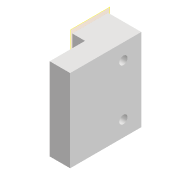
# Autodesk Inventor part: 30_XYTable_Aliexpress_Translatorarm_y
Saved by Autodesk Inventor 2022 (Build 260153000, 153)
## iProperties
Created: 2022-10-26
Part Number: 30_XYTable_Aliexpress_Translatorarm_y
Material: Generisch
Document SubType Name: Modeling
Designer: diederichbenedict
Density: 1 g/cm^3
Appearance: Vorgabe
Author: diederichbenedict
Autodesk Inventor part; units mm, degrees
ref_plane "YZ Plane" through (0, 0, 0) normal (1, 0, 0) x (0, 1, 0)
ref_plane "XZ Plane" through (0, 0, 0) normal (0, 1, 0) x (-1, 0, 0)
ref_plane "XY Plane" through (0, 0, 0) normal (0, 0, 1) x (1, 0, 0)
ref_plane "Arbeitsebene2" through (35, 26.0506, 0) normal (1, 0, 0) x (0, 0, -1)
sketch "Skizze6" plane through (35, 26.0506, 0) normal (1, 0, 0) x (0, 0, -1)
  line L0 (-14, 32.2) -> (-14, 0) projected
  line L1 (0, 0) -> (-14, 0) projected
  line L2 (0, 32.2) -> (0, 0) projected
  line L3 (0, 32.2) -> (-14, 32.2) projected
  line L4 (-8.5, 27.35) -> (0, 27.35)
  line L5 (-8.5, 24.85) -> (0, 24.85)
  line L6 (-8.5, 7.35) -> (0, 7.35)
  line L7 (-8.5, 4.85) -> (0, 4.85)
  circle A0 centre (-7, 26.1) radius 1.6
  circle A1 centre (-7, 6.1) radius 1.6
  point P0 (0, -26.0506)
  dimension "d40" = 3.2
  dimension "d41" = 3.2
  dimension "d42" = 1.25
  dimension "d43" = 1.25
  dimension "d44" = 7
  dimension "d45" = 7
  constraints: 8 end point, 4 horizontal, 2 centre point, 8 other
  measures "d40" diameter of A0
  measures "d41" diameter of A1
  measures "d42" distance from line of L6 A1.centre
  measures "d43" distance from line of A0.centre L4
  measures "d44" distance from line of A0.centre L0
  measures "d45" distance from line of L0 A1.centre
extrude "Extrusion6" add sketch "Skizze6" along normal blind 5 contours L3 L2 L4 A0 L5 L6 A1 L7 L1 L0 | L2 L5 A0 L4 | L7 A1 L6 L2
sketch "Skizze7" plane through (40, 26.0506, 0) normal (1, 0, 0) x (0, 0, -1)
  line L0 (0, 32.2) -> (-14, 32.2) projected
  line L1 (-14, 32.2) -> (-14, 0) projected
  line L2 (-14, 0) -> (0, 0) projected
  line L3 (0, 0) -> (0, 32.2) projected
  circle A0 centre (-7, 26.1) radius 1.6 projected
  circle A1 centre (-7, 6.1) radius 1.6 projected
  line L4 (-58.75, 26.0265) -> (-58.75, 86.0265) projected
  line L5 (0, 32.2) -> (-27.8, 32.2)
  line L6 (-27.8, 32.2) -> (-27.8, 0)
  line L7 (-27.8, 0) -> (0, 0)
  line L8 (0, 0) -> (0, 32.2)
  line L9 (0, 32.2) -> (-14, 32.2) projected
  line L10 (0, 32.2) -> (-27.8, 32.2)
  line L11 (-27.8, 32.2) -> (-27.8, 52.2)
  line L12 (-27.8, 52.2) -> (0, 52.2)
  line L13 (0, 52.2) -> (0, 32.2)
  point P0 (0, -26.0506)
  point P1 (-14, 0)
  point P2 (-14, 32.2)
  dimension "d48" = 27.8
  dimension "d51" = 20
  constraints: 16 end point, 4 parallel, 2 horizontal, 2 perpendicular
  measures "d48" distance of L7.end L6.end
  measures "d51" distance of L10.end L11.end
extrude "Extrusion7" add sketch "Skizze7" along normal blind 8
sketch "Skizze8" plane through (35, 26.0506, 0) normal (0, 0, -1) x (-1, 0, 0)
  line L0 (-13, 24.5) -> (0, 24.5) projected
  line L1 (-13, 27.7) -> (0, 27.7) projected
  line L2 (-13, 7.7) -> (0, 7.7) projected
  line L3 (-13, 4.5) -> (0, 4.5) projected
  line L4 (0, 0) -> (0, 32.2) projected
  line L5 (0, 32.2) -> (-5, 32.2) projected
  line L6 (-5, 32.2) -> (-5, 52.2) projected
  line L7 (-5, 52.2) -> (-13, 52.2) projected
  line L8 (-13, 0) -> (-13, 52.2) projected
  line L9 (0, 0) -> (-13, 0) projected
  circle A0 centre (-9.5, 39.8052) radius 1.6 construction
  circle A1 centre (-9.5, 13.7) radius 1.4 construction
  circle A2 centre (-9.5, 29.7) radius 1.4 construction
  circle A3 centre (-9.5, 45.7) radius 1.4 construction
  point P0 (35, -26.0506)
  dimension "d52" = 2.8
  dimension "d53" = 3.5
  dimension "d54" = 6
  dimension "d55" = 2.8
  dimension "d56" = 16
  dimension "d57" = 2.8
  dimension "d58" = 16
  constraints: 3 centre point
  measures "d52" diameter of A1
  measures "d53" distance from line of A1.centre L8
  measures "d54" distance from line of A1.centre L2
  measures "d55" diameter of A2
  measures "d56" distance of A1.centre A2.centre
  measures "d57" diameter of A3
  measures "d58" distance of A2.centre A3.centre
hole "Bohrung1" at (44.5, 39.7506, 0) at (44.5, 55.7506, 0) at (44.5, 71.7506, 0) direction (0, 0, 1) diameter 3.2 end through all counterbore diameter 6.5 counterbore depth 20
chamfer "Fase4" distance 10 angle 45 1 edges at (48, 52.1506, 0)
sketch "Skizze9" plane through (48, 26.0506, 0) normal (1, 0, 0) x (0, 0, -1)
  circle A0 centre (-7, 6.1) radius 1.6 projected
  arc A1 (-8.3185, 27.0064) -> (-5.4844, 26.6128) centre (-7, 26.1) ccw projected
  point P0 (0, -26.0506)
hole "Bohrung2" at (48, 32.1506, 7) at (48, 52.1506, 7) direction (-1, 0, 0) diameter 3.2 end through all counterbore diameter 6.5 counterbore depth 7
